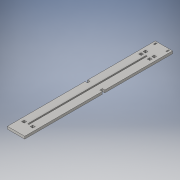
# Autodesk Inventor part: Arm Base
Saved by Autodesk Inventor 2016 (Build 200138000, 138)
## iProperties
Created: 2016-04-23
Part Number: Arm Base
Material: Generic
Document SubType Name: Modeling
Designer: rubenjm
Density: 1 g/cm^3
Appearance: Default
Author: rubenjm
Autodesk Inventor part; units mm, degrees
ref_plane "YZ Plane" through (0, 0, 0) normal (1, 0, 0) x (0, 1, 0)
ref_plane "XZ Plane" through (0, 0, 0) normal (0, 1, 0) x (-1, 0, 0)
ref_plane "XY Plane" through (0, 0, 0) normal (0, 0, 1) x (1, 0, 0)
sketch "Sketch1" plane through (0, 0, 0) normal (0, 1, 0) x (-1, 0, 0)
  line L0 (0, 0) -> (88.9, 0)
  line L1 (88.9, -762) -> (0, -762)
  line L2 (0, -762) -> (0, 0)
  line L3 (88.9, 0) -> (0, 0) construction
  line L4 (0, 0) -> (0, -50.8) construction
  line L5 (88.9, 0) -> (88.9, -762)
  dimension "d0" = 88.9
  dimension "d3" = 50.8
  dimension "d47" = 762
  constraints: 12 end point, 2 horizontal, 2 parallel, 2 perpendicular
  measures "d0" distance of L1.start L1.end
  measures "d3" distance of L4.end L3.end
  measures "d47" distance of L1.end L0.start
extrude "Extrusion3" add sketch "Sketch1" along normal blind 12.7
sketch "Sketch2" plane through (0, 12.7, 0) normal (0, 1, 0) x (1, 0, 0)
  line L0 (0, 762) -> (-88.9, 762) construction
  line L1 (-44.45, 762) -> (666.75, 762) construction
  line L2 (-41.275, 63.5) -> (-47.625, 63.5)
  line L3 (-47.625, 63.5) -> (-47.625, 673.1)
  line L4 (-47.625, 673.1) -> (-41.275, 673.1)
  line L5 (-41.275, 673.1) -> (-41.275, 63.5)
  line L6 (-44.45, 63.5) -> (-44.45, 0) construction
  line L7 (-88.9, 0) -> (0, 0) construction
  dimension "d21" = 6.35
  dimension "d22" = 609.6
  dimension "d25" = 63.5
  constraints: 12 end point, 3 midpoint, 2 horizontal, 2 parallel, 1 perpendicular
  measures "d21" distance of L3.end L4.end
  measures "d22" distance of L2.end L3.end
  measures "d25" distance of L6.start L6.end
extrude "Extrusion4" cut sketch "Sketch2" against normal through all
sketch "Sketch3" plane through (0, 0, 0) normal (0, -1, 0) x (1, 0, 0)
  line L0 (-41.275, -673.1) -> (-41.275, -63.5) construction
  line L1 (-41.275, -63.5) -> (-22.225, -63.5) construction
  line L2 (-47.625, -63.5) -> (-41.275, -63.5) construction
  line L3 (-44.45, -63.5) -> (-44.45, 0) construction
  line L4 (-47.625, -63.5) -> (-66.675, -63.5) construction
  line L5 (-28.575, -57.15) -> (-15.875, -57.15)
  line L6 (-15.875, -57.15) -> (-15.875, -69.85)
  line L7 (-15.875, -69.85) -> (-28.575, -69.85)
  line L8 (-28.575, -69.85) -> (-28.575, -57.15)
  line L9 (-28.575, -57.15) -> (-15.875, -69.85) construction
  line L10 (-15.875, -57.15) -> (-28.575, -69.85) construction
  line L11 (-60.325, -57.15) -> (-73.025, -57.15)
  line L12 (-73.025, -57.15) -> (-73.025, -69.85)
  line L13 (-73.025, -69.85) -> (-60.325, -69.85)
  line L14 (-60.325, -69.85) -> (-60.325, -57.15)
  line L15 (-60.325, -57.15) -> (-73.025, -69.85) construction
  line L16 (-73.025, -57.15) -> (-60.325, -69.85) construction
  line L17 (-28.575, -660.4) -> (-15.875, -660.4)
  line L18 (-15.875, -660.4) -> (-15.875, -673.1)
  line L19 (-15.875, -673.1) -> (-28.575, -673.1)
  line L20 (-28.575, -673.1) -> (-28.575, -660.4)
  line L21 (-28.575, -660.4) -> (-15.875, -673.1) construction
  line L22 (-15.875, -660.4) -> (-28.575, -673.1) construction
  line L23 (-60.325, -660.4) -> (-73.025, -660.4)
  line L24 (-73.025, -660.4) -> (-73.025, -673.1)
  line L25 (-73.025, -673.1) -> (-60.325, -673.1)
  line L26 (-60.325, -673.1) -> (-60.325, -660.4)
  line L27 (-60.325, -660.4) -> (-73.025, -673.1) construction
  line L28 (-73.025, -660.4) -> (-60.325, -673.1) construction
  line L29 (-47.625, -673.1) -> (-41.275, -673.1) construction
  line L30 (-28.575, -673.1) -> (-60.325, -673.1) construction
  line L31 (-44.45, -673.1) -> (-44.45, -695.706) construction
  line L32 (-44.45, -673.1) -> (-21.844, -673.1) construction
  line L33 (-28.575, -695.706) -> (-28.575, -683.006)
  line L34 (-15.875, -695.706) -> (-28.575, -695.706)
  line L35 (-15.875, -683.006) -> (-15.875, -695.706)
  line L36 (-15.875, -683.006) -> (-28.575, -695.706) construction
  line L37 (-28.575, -683.006) -> (-15.875, -683.006)
  line L38 (-28.575, -683.006) -> (-15.875, -695.706) construction
  line L39 (-60.325, -695.706) -> (-60.325, -683.006)
  line L40 (-60.325, -683.006) -> (-73.025, -683.006)
  line L41 (-73.025, -683.006) -> (-73.025, -695.706)
  line L42 (-60.325, -683.006) -> (-73.025, -695.706) construction
  line L43 (-73.025, -683.006) -> (-60.325, -695.706) construction
  line L44 (-73.025, -695.706) -> (-60.325, -695.706)
  line L45 (-28.575, -695.706) -> (-60.325, -695.706) construction
  line L46 (0, -762) -> (-88.9, -762) construction
  line L47 (-44.45, -762) -> (-44.45, -755.65) construction
  line L48 (-44.45, -755.65) -> (-15.875, -755.65) construction
  line L49 (-15.875, -755.65) -> (-9.525, -755.65)
  line L50 (-9.525, -755.65) -> (-9.525, -742.95)
  line L51 (-9.525, -742.95) -> (-15.875, -742.95)
  line L52 (-15.875, -742.95) -> (-15.875, -755.65)
  line L53 (-73.025, -755.65) -> (-79.375, -755.65)
  line L54 (-79.375, -755.65) -> (-79.375, -742.95)
  line L55 (-79.375, -742.95) -> (-73.025, -742.95)
  line L56 (-73.025, -742.95) -> (-73.025, -755.65)
  point P0 (0, 0)
  point P1 (-22.225, -666.75)
  point P2 (-66.675, -666.75)
  point P3 (-22.225, -689.356)
  point P4 (-66.675, -689.356)
  point P5 (-21.844, -695.706)
  dimension "d26" = 19.05
  dimension "d27" = 12.7
  dimension "d28" = 12.7
  dimension "d29" = 12.7
  dimension "d30" = 12.7
  dimension "d33" = 12.7
  dimension "d34" = 12.7
  dimension "d35" = 12.7
  dimension "d36" = 12.7
  dimension "d37" = 22.606
  dimension "d38" = 90
  dimension "d39" = 12.7
  dimension "d40" = 12.7
  dimension "d41" = 12.7
  dimension "d42" = 12.7
  dimension "d43" = 6.35
  dimension "d44" = 28.575
  dimension "d45" = 6.35
  dimension "d46" = 12.7
  constraints: 106 end point, 15 midpoint, 14 parallel, 9 horizontal, 9 perpendicular, 5 symmetric about line, 3 vertical, 2 collinear
  measures "d26" distance of L0.end L1.end
  measures "d27" distance of L6.end L7.end
  measures "d28" distance of L5.end L6.end
  measures "d29" distance of L13.end L12.end
  measures "d30" distance of L12.end L11.end
  measures "d33" distance of L19.start L20.start
  measures "d34" distance of L18.start L19.start
  measures "d35" distance of L26.start L24.end
  measures "d36" distance of L24.end L23.end
  measures "d37" distance of L31.start L31.end
  measures "d38" angle of L31 L32
  measures "d39" distance of L34.start L33.start
  measures "d40" distance of L37.end L34.start
  measures "d41" distance of L44.end L41.end
  measures "d42" distance of L41.end L41.start
  measures "d43" distance of L47.start L47.end
  measures "d44" distance of L47.end L48.end
  measures "d45" distance of L51.end L50.end
  measures "d46" distance of L50.end L49.end
extrude "Extrusion5" cut sketch "Sketch3" against normal through all
sketch "Sketch4" plane through (0, 0, 0) normal (0, -1, 0) x (1, 0, 0)
  line L0 (-88.9, -406.4) -> (0, -406.4) construction
  line L1 (-88.9, -400.05) -> (-76.2, -400.05)
  line L2 (-76.2, -400.05) -> (-76.2, -412.75)
  line L3 (-76.2, -412.75) -> (-88.9, -412.75)
  line L4 (-88.9, -400.05) -> (-88.9, -412.75)
  line L5 (0, -400.05) -> (-12.7, -400.05)
  line L6 (-12.7, -400.05) -> (-12.7, -412.75)
  line L7 (-12.7, -412.75) -> (0, -412.75)
  line L8 (0, -400.05) -> (0, -412.75)
  line L9 (-15.875, -742.95) -> (-15.875, -755.65) construction
  line L10 (-79.375, -755.65) -> (-73.025, -755.65) construction
  line L11 (-15.875, -755.65) -> (-73.025, -755.65) construction
  line L12 (-28.575, -69.85) -> (-28.575, -57.15) construction
  line L13 (-28.575, -57.15) -> (-60.325, -57.15) construction
  line L14 (-44.45, -57.15) -> (-44.45, -755.65) construction
  point P0 (-44.45, -406.4)
  dimension "d49" = 12.7
  dimension "d52" = 12.7
  constraints: 24 end point, 6 midpoint, 4 horizontal, 1 parallel, 1 perpendicular
  measures "d49" distance of L1.end L2.end
  measures "d52" distance of L2.end L3.end
extrude "Extrusion6" cut sketch "Sketch4" against normal through all
body "Solid3"
